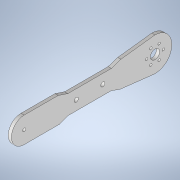
# Autodesk Inventor part: Brazo1Izquierda
Saved by Autodesk Inventor 2022 (Build 260153000, 153)
## iProperties
Created: 2021-09-13
Part Number: Brazo1Izquierda
Material: Generic
Document SubType Name: Modeling
Designer: Administrador
Density: 1 g/cm^3
Appearance: Default
Author: Administrador
Autodesk Inventor part; units mm, degrees
ref_plane "YZ Plane" through (0, 0, 0) normal (1, 0, 0) x (0, 1, 0)
ref_plane "XZ Plane" through (0, 0, 0) normal (0, 1, 0) x (-1, 0, 0)
ref_plane "XY Plane" through (0, 0, 0) normal (0, 0, 1) x (1, 0, 0)
sketch "Sketch1" plane through (0, 0, 0) normal (1, 0, 0) x (0, 1, 0)
  circle A0 centre (12, -104.7) radius 4.375
  circle A1 centre (12, -104.7) radius 9 construction
  line L0 (12, -116.7) -> (12, -104.7) construction
  line L1 (12, -113.7) -> (12, -112.5)
  circle A2 centre (12, -112.5) radius 1.2
  circle A3 centre (12, -55.7) radius 2
  circle A4 centre (18.755, -108.6) radius 1.2
  circle A5 centre (18.755, -100.8) radius 1.2
  circle A6 centre (12, -96.9) radius 1.2
  circle A7 centre (5.245, -100.8) radius 1.2
  circle A8 centre (5.245, -108.6) radius 1.2
  line L2 (3, -43.2) -> (21, -43.2) construction
  line L3 (12, -116.7) -> (12, -71.7) construction
  line L4 (12, -71.7) -> (12, -63.7) construction
  line L5 (12, -63.7) -> (21, -63.7) construction
  line L6 (12, -63.7) -> (3, -63.7) construction
  line L7 (24, -72.7) -> (21, -63.7)
  line L8 (0, -71.7) -> (3, -63.7)
  line L9 (3, -43.2) -> (3, -63.7)
  line L10 (21, -43.2) -> (21, -63.7)
  circle A9 centre (12, -30.7) radius 2
  line L11 (24, -13.7) -> (21, -22.7)
  line L12 (0, -14.7) -> (3, -22.7)
  line L13 (12, -14.7) -> (12, -22.7) construction
  line L14 (12, -22.7) -> (3, -22.7) construction
  line L15 (3, -43.2) -> (3, -22.7)
  line L16 (21, -43.2) -> (21, -22.7)
  line L17 (12, -22.7) -> (21, -22.7) construction
  circle A10 centre (12, 18.3) radius 1.5
  arc A11 (-3.3865, -101.1088) -> (27.3606, -100.9997) centre (12, -104.7) ccw
  arc A12 (-3.3865, -101.1088) -> (27.3606, -100.9997) centre (12, -104.7) ccw
  line L18 (0, -71.7) -> (-3.8, -104.7)
  line L19 (24, -72.7) -> (27.8, -104.7)
  arc A13 (24, 18.3) -> (0, 18.3) centre (12, 18.3) ccw
  line L20 (0, -14.7) -> (0, 18.3)
  line L21 (24, -13.7) -> (24, 18.3)
  point P0 (0, 0)
  point P1 (1.5, 26.1095)
  point P2 (22.5, 26.1095)
  point P3 (19.7942, -109.2)
  point P4 (19.7942, -100.2)
  point P5 (12, -95.7)
  point P6 (4.2058, -100.2)
  point P7 (4.2058, -109.2)
  dimension "d4" = 18
  dimension "d3" = 8.75
  dimension "d5" = 1.2
  dimension "d6" = 4
  dimension "d7" = 360
  dimension "d8" = 45
  dimension "d9" = 8
  dimension "d10" = 9
  dimension "d11" = 9
  dimension "d13" = 8
  dimension "d14" = 12.5
  dimension "d15" = 3
  dimension "d19" = 24
  constraints: 44 end point, 8 point on circle, 7 centre point, 7 symmetric about line, 4 point on line, 4 vertical, 3 coincident, 3 horizontal, 3 vertical alignment, 2 tangent, 1 concentric, 1 perpendicular, 40 other
  measures "d3" diameter of A0
  measures "d5" distance of L1.start L1.end
  measures "d6" diameter of A3
  measures "d8" distance of L0.start L3.end
  measures "d9" distance of L3.end L4.end
  measures "d10" distance of L4.end L5.end
  measures "d11" distance of L4.end L6.end
  measures "d13" distance of A3.centre L4.end
  measures "d14" distance from line of L2 A3.centre
  measures "d15" diameter of A10
  measures "d19" diameter of A13
extrude "Extrusion1" add sketch "Sketch1" along normal blind 3 contours L19 A11 L18 L8 L9 L15 L12 L20 A13 L21 L11 L16 L10 L7
body "Solid1"
